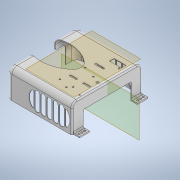
# Autodesk Inventor part: Enclosure
Saved by Autodesk Inventor 2020 (Build 240168000, 168)
## iProperties
Created: 2020-02-08
Part Number: Enclosure
Material: Generic
Document SubType Name: Modeling
Designer: pp445
Density: 1 g/cm^3
Appearance: Default
Author: pp445
Autodesk Inventor part; units mm, degrees
ref_plane "YZ Plane" through (0, 0, 0) normal (1, 0, 0) x (0, 1, 0)
ref_plane "XZ Plane" through (0, 0, 0) normal (0, 1, 0) x (-1, 0, 0)
ref_plane "XY Plane" through (0, 0, 0) normal (0, 0, 1) x (1, 0, 0)
sketch "Sketch1" plane through (0, 0, 0) normal (0, 1, 0) x (-1, 0, 0)
  line L0 (0, 0) -> (81, 0)
  line L1 (81, 0) -> (81, -120)
  line L2 (81, -120) -> (0, -120)
  line L3 (0, -120) -> (0, 0)
  line L4 (217, 28.5) -> (81, 28.5)
  line L5 (81, 28.5) -> (81, -146)
  line L6 (81, -146) -> (217, -146)
  line L7 (217, -146) -> (217, 28.5)
  line L8 (81, -60) -> (0, -60) construction
  point P0 (81, 0)
  point P1 (81, -120)
  dimension "d0" = 120
  dimension "d1" = 81
  dimension "d2" = 174.5
  dimension "d4" = 136
  dimension "d40" = 26
  constraints: 18 end point, 4 parallel, 2 horizontal, 2 perpendicular, 1 collinear, 1 midpoint, 1 point on line
  measures "d0" distance of L2.end L0.start
  measures "d1" distance of L0.start L0.end
  measures "d2" distance between parallel lines of L6 L4
  measures "d4" distance of L4.start L4.end
  measures "d40" distance between parallel lines of L2 L6
extrude "Extrusion1" add sketch "Sketch1" against normal blind 70
shell "Shell1" thickness 1.25 removed faces 3 at (-171.6667, -70, -39.1667) at (0, -23.3333, -40) at (-217, -23.3333, -87.8333)
sketch "Sketch3" plane through (0, -70, 0) normal (0, -1, 0) x (1, 0, 0)
  line L0 (-81, -146) -> (-81, -120) projected
  line L1 (0, -1.25) -> (0, 0) projected
  line L2 (0, 0) -> (-81, 0)
  line L3 (-81, -120) -> (0, -120) projected
  line L4 (0, -120) -> (-81, -120)
  line L5 (-81, -120) -> (-81, -146)
  line L6 (-81, -146) -> (0, -146)
  line L7 (0, -146) -> (0, -120)
  line L8 (-81, 0) -> (-81, 28.5) projected
  line L9 (-81, 0) -> (0, 0) projected
  line L10 (-217, 28.5) -> (-81, 28.5) projected
  line L11 (0, 0) -> (-81, 0)
  line L12 (-81, 0) -> (-81, 28.5)
  line L13 (-81, 28.5) -> (0, 28.5)
  line L14 (0, 28.5) -> (0, 0)
  constraints: 18 end point, 4 parallel, 3 horizontal, 2 perpendicular
extrude "Extrusion3" add sketch "Sketch3" against normal blind 3.175
sketch "Sketch5" plane through (0, -66.825, 0) normal (0, 1, 0) x (1, 0, 0)
  line L0 (0, 120) -> (0, 146) projected
  line L1 (0, 146) -> (-81, 146) projected
  line L2 (-81, 120) -> (-81, 146) projected
  line L3 (0, 120) -> (-81, 120) projected
  line L4 (-81, 0) -> (0, 0) projected
  line L5 (-81, -28.5) -> (-81, 0) projected
  line L6 (-81, -28.5) -> (0, -28.5) projected
  line L7 (0, -28.5) -> (0, 0) projected
  line L8 (0, 146) -> (0, 118.75) projected
  line L9 (-81, 120) -> (-81, 146) projected
  line L10 (0, 1.25) -> (0, -28.5) projected
  line L11 (0, -14.25) -> (-81, -14.25) construction
  line L12 (-81, -28.5) -> (-81, 0) projected
  circle A0 centre (-20.7, -14.25) radius 2.3813
  circle A1 centre (-46.1, -14.25) radius 2.3813
  circle A2 centre (-71.5, -14.25) radius 2.3813
  circle A3 centre (-20.7, 133.3) radius 2.3813
  circle A4 centre (-46.1, 133.3) radius 2.3813
  circle A5 centre (-71.5, 133.3) radius 2.3813
  line L13 (-81, 133.3) -> (0, 133.3) construction
  dimension "d18" = 20.7
  dimension "d19" = 25.4
  dimension "d20" = 25.4
  dimension "d21" = 4.7625
  dimension "d22" = 4.7625
  dimension "d23" = 4.7625
  dimension "d41" = 4.7625
  dimension "d42" = 4.7625
  dimension "d43" = 4.7625
  dimension "d44" = 20.7
  dimension "d45" = 25.4
  dimension "d46" = 25.4
  dimension "d47" = 13.3
  constraints: 9 point on line, 6 centre point, 4 end point, 1 midpoint, 1 perpendicular
  measures "d18" distance from line of L7 A0.centre
  measures "d19" distance of A0.centre A1.centre
  measures "d20" distance of A1.centre A2.centre
  measures "d21" diameter of A0
  measures "d22" diameter of A1
  measures "d23" diameter of A2
  measures "d41" diameter of A3
  measures "d42" diameter of A4
  measures "d43" diameter of A5
  measures "d44" distance from line of L8 A3.centre
  measures "d45" distance of A3.centre A4.centre
  measures "d46" distance of A4.centre A5.centre
  measures "d47" distance between parallel lines of L3 L13
extrude "Extrusion4" cut sketch "Sketch5" against normal up to surface (3.175 mm away) contours A3 | A4 | A5
ref_plane "Work Plane1" through (0, -1.25, -60) normal (0, 0, -1) x (-1, 0, 0)
mirror "Mirror1" about plane through (0, -1.25, -60) normal (0, 0, -1) of "Extrusion4"
mirror "Mirror2" about plane through (0, -1.25, -60) normal (0, 0, -1) of "Extrusion4"
sketch "Sketch9" plane through (0, 0, 0) normal (1, 0, 0) x (0, 0, -1)
  line L0 (1.25, -70) -> (1.25, -1.25) projected
  line L1 (1.25, -1.25) -> (118.75, -1.25) projected
  line L2 (118.75, -1.25) -> (118.75, -70) projected
  line L3 (146, -70) -> (118.75, -70) projected
  line L4 (146, -70) -> (146, -66.825) projected
  line L5 (120, -66.825) -> (146, -66.825) projected
  line L6 (120, 0) -> (120, -66.825) projected
  line L7 (0, 0) -> (120, 0) projected
  line L8 (0, 0) -> (0, -66.825) projected
  line L9 (-28.5, -66.825) -> (0, -66.825) projected
  line L10 (-28.5, -70) -> (-28.5, -66.825) projected
  line L11 (1.25, -70) -> (-28.5, -70) projected
extrude "Extrusion8" cut sketch "Sketch9" against normal blind 10
sketch "Sketch10" plane through (-10, 0, 0) normal (1, 0, 0) x (0, 0, -1)
  line L0 (1.25, -70) -> (-28.5, -70) projected
  line L1 (1.25, -1.25) -> (1.25, -70) projected
  line L2 (118.75, -1.25) -> (1.25, -1.25) projected
  line L3 (118.75, -70) -> (118.75, -1.25) projected
  line L4 (146, -70) -> (118.75, -70) projected
  line L5 (146, -66.825) -> (146, -70) projected
  line L6 (120, -66.825) -> (146, -66.825) projected
  line L7 (120, 0) -> (120, -66.825) projected
  line L8 (0, 0) -> (120, 0) projected
  line L9 (0, -66.825) -> (0, 0) projected
  line L10 (-28.5, -66.825) -> (0, -66.825) projected
  line L11 (-28.5, -70) -> (-28.5, -66.825) projected
  line L12 (1.25, -70) -> (-28.5, -70) projected
  line L13 (-28.5, -66.825) -> (-24.5, -66.825)
  line L14 (-24.5, -66.825) -> (-24.5, -70)
  line L15 (-24.5, -70) -> (-28.5, -70)
  line L16 (-28.5, -70) -> (-28.5, -66.825)
  dimension "d50" = 4
  constraints: 8 end point, 2 parallel, 1 horizontal, 1 perpendicular, 1 point on line
  measures "d50" distance between parallel lines of L11 L14
extrude "Extrusion9" cut sketch "Sketch10" against normal up to surface (71 mm away) contours L0 L11 L10 L14
pattern_linear "Rectangular Pattern2" count 2 spacing 7 along (0, 0, -1) count 2 spacing 7 along (0, 0, 1) of "Extrusion4"
mirror "Mirror3" about plane through (0, -1.25, -60) normal (0, 0, -1) of "Extrusion4", "Rectangular Pattern2"
sketch "Sketch11" plane through (-81, -70, 28.5) normal (0, 0, 1) x (1, 0, 0)
  line L0 (0, 70) -> (0, 0) projected
  line L1 (-136, 70) -> (0, 70) projected
  line L2 (0, 0) -> (-136, 0) projected
  line L3 (-1.25, 0) -> (-114, 0) projected
  line L4 (-3.175, 0) -> (-109.175, 0)
  line L5 (-109.175, 0) -> (-109.175, 58.175)
  line L6 (-109.175, 58.175) -> (-3.175, 58.175)
  line L7 (-3.175, 58.175) -> (-3.175, 0)
  line L8 (-95.5478, 52.5) -> (-95.5478, 7.5)
  circle A0 centre (-79.7364, 30) radius 27.5 construction
  arc A1 (-95.5478, 52.5) -> (-95.5478, 7.5) centre (-79.7364, 30) ccw
  line L9 (-56.175, 58.175) -> (-56.175, 0) construction
  line L10 (-16.8022, 52.5) -> (-16.8022, 7.5)
  circle A2 centre (-32.6136, 30) radius 27.5 construction
  arc A3 (-16.8022, 7.5) -> (-16.8022, 52.5) centre (-32.6136, 30) ccw
  line L11 (-79.7364, 30) -> (-32.6136, 30) construction
  line L12 (-93.0078, 54) -> (-80.3078, 54)
  line L13 (-80.3078, 54) -> (-80.3078, 6)
  line L14 (-80.3078, 6) -> (-93.0078, 6)
  line L15 (-93.0078, 6) -> (-93.0078, 54)
  line L16 (-93.0078, 30) -> (-80.3078, 30) construction
  line L17 (-77.7678, 54) -> (-65.0678, 54)
  line L18 (-65.0678, 54) -> (-65.0678, 6)
  line L19 (-65.0678, 6) -> (-77.7678, 6)
  line L20 (-77.7678, 6) -> (-77.7678, 54)
  line L21 (-62.5278, 54) -> (-49.8278, 54)
  line L22 (-49.8278, 54) -> (-49.8278, 6)
  line L23 (-49.8278, 6) -> (-62.5278, 6)
  line L24 (-62.5278, 6) -> (-62.5278, 54)
  line L25 (-47.2878, 54) -> (-34.5878, 54)
  line L26 (-34.5878, 54) -> (-34.5878, 6)
  line L27 (-34.5878, 6) -> (-47.2878, 6)
  line L28 (-47.2878, 6) -> (-47.2878, 54)
  line L29 (-32.0478, 54) -> (-19.3478, 54)
  line L30 (-19.3478, 54) -> (-19.3478, 6)
  line L31 (-19.3478, 6) -> (-32.0478, 6)
  line L32 (-32.0478, 6) -> (-32.0478, 54)
  line L33 (-136, 70) -> (-136, 0) projected
  point P0 (81, 70)
  point P1 (-65.0678, 30)
  point P2 (-77.7678, 30)
  point P3 (-49.8278, 30)
  point P4 (-62.5278, 30)
  point P5 (-34.5878, 30)
  point P6 (-47.2878, 30)
  point P7 (-19.3478, 30)
  point P8 (-32.0478, 30)
  dimension "d59" = 3.175
  dimension "d60" = 106
  dimension "d61" = 58.175
  dimension "d62" = 45
  dimension "d63" = 55
  dimension "d64" = 30
  dimension "d66" = 29.4386
  dimension "d70" = 48
  dimension "d71" = 2.54
  dimension "d72" = 12.7
  dimension "d83" = 15.24
  constraints: 58 end point, 8 point on circle, 4 centre point, 4 horizontal, 4 midpoint, 4 parallel, 4 symmetric about line, 3 perpendicular, 2 coincident, 1 collinear, 1 point on line, 1 vertical, 42 other
  measures "d59" distance between parallel lines of L0 L7
  measures "d60" distance of L5.end L6.end
  measures "d61" distance of L4.end L5.end
  measures "d62" distance of L8.start L8.end
  measures "d63" diameter of A0
  measures "d64" distance from line of L2 A0.centre
  measures "d66" distance from line of L5 A0.centre
  measures "d70" distance of L12.end L13.end
  measures "d71" distance between parallel lines of L8 L15
  measures "d72" distance between parallel lines of L15 L13
  measures "d83" distance of L12.start L17.start
extrude "Extrusion10" cut sketch "Sketch11" against normal up to surface (174.5 mm away) contours L8 A1 | A3 L10 | L12 L13 L14 L15 | L17 L18 L19 L20 | L21 L22 L23 L24 | L25 L26 L27 L28 | L29 L30 L31 L32
fillet "Fillet1" radius 2.54 8 edges at (-176.5478, -17.5, 27.875) (-176.5478, -62.5, 27.875) (-97.8022, -17.5, 27.875) (-97.8022, -62.5, 27.875) (-97.8022, -17.5, -145.375) (-97.8022, -62.5, -145.375) (-176.5478, -62.5, -145.375) (-176.5478, -17.5, -145.375)
fillet "Fillet2" radius 6.35 40 edges at (-174.0078, -64, 27.875) (-161.3078, -64, 27.875) (-161.3078, -16, 27.875) (-174.0078, -16, 27.875) (-158.7678, -64, 27.875) (-143.5278, -64, 27.875) (-128.2878, -64, 27.875) (-113.0478, -64, 27.875) (-100.3478, -64, 27.875) (-115.5878, -64, 27.875) (-130.8278, -64, 27.875) (-146.0678, -64, 27.875) (-158.7678, -16, 27.875) (-143.5278, -16, 27.875) (-128.2878, -16, 27.875) (-113.0478, -16, 27.875) (-100.3478, -16, 27.875) (-115.5878, -16, 27.875) (-130.8278, -16, 27.875) (-146.0678, -16, 27.875) (-174.0078, -16, -145.375) (-158.7678, -16, -145.375) (-143.5278, -16, -145.375) (-128.2878, -16, -145.375) (-113.0478, -16, -145.375) (-100.3478, -16, -145.375) (-115.5878, -16, -145.375) (-130.8278, -16, -145.375) (-146.0678, -16, -145.375) (-161.3078, -16, -145.375) (-100.3478, -64, -145.375) (-115.5878, -64, -145.375) (-130.8278, -64, -145.375) (-146.0678, -64, -145.375) (-161.3078, -64, -145.375) (-174.0078, -64, -145.375) (-158.7678, -64, -145.375) (-143.5278, -64, -145.375) (-128.2878, -64, -145.375) (-113.0478, -64, -145.375)
sketch "Sketch12" plane through (-10, 0, 0) normal (1, 0, 0) x (0, 0, -1)
  line L0 (-24.5, -66.825) -> (-24.5, -70) projected
  line L1 (1.25, -70) -> (-24.5, -70) projected
  line L2 (1.25, -1.25) -> (1.25, -70) projected
  line L3 (118.75, -1.25) -> (1.25, -1.25) projected
  line L4 (118.75, -70) -> (118.75, -1.25) projected
  line L5 (146, -70) -> (118.75, -70) projected
  line L6 (146, -66.825) -> (146, -70) projected
  line L7 (120, -66.825) -> (146, -66.825) projected
  line L8 (120, 0) -> (120, -66.825) projected
  line L9 (0, 0) -> (120, 0) projected
  line L10 (0, -66.825) -> (0, 0) projected
  line L11 (-24.5, -66.825) -> (0, -66.825) projected
  line L12 (0, -66.825) -> (0, 0) projected
  line L13 (1.25, -70) -> (0, -70)
  line L14 (0, -70) -> (0, 0)
  line L15 (0, 0) -> (1.25, 0)
  line L16 (1.25, 0) -> (1.25, -70)
  line L17 (118.75, -70) -> (144.75, -70) projected
  line L18 (120, 0) -> (120, -66.825) projected
  line L19 (118.75, -70) -> (120, -70)
  line L20 (120, -70) -> (120, 0)
  line L21 (120, 0) -> (118.75, 0)
  line L22 (118.75, 0) -> (118.75, -70)
  line L23 (118.75, 0) -> (1.25, 0)
  line L24 (1.25, 0) -> (1.25, -1.25)
  line L25 (1.25, -1.25) -> (118.75, -1.25)
  line L26 (118.75, -1.25) -> (118.75, 0)
  constraints: 24 end point, 6 parallel, 3 horizontal, 3 perpendicular
extrude "Extrusion11" cut sketch "Sketch12" against normal up to surface (72.25 mm away) contours L10 L9 L16 L2 L1 L14 | L9 L22 L3 L16 | L9 L8 L20 L5 L4 L22
sketch "Sketch13" plane through (-82.25, -1.25, -120) normal (1, 0, 0) x (0, 0, -1)
  line L0 (-120, 1.25) -> (0, 1.25) projected
  line L1 (-120, 0) -> (0, 0) projected
  line L2 (0, 1.25) -> (0, 0) projected
  line L3 (-120, 1.25) -> (0, 1.25) projected
  line L4 (-120, 0) -> (-120, 1.25) projected
  line L5 (0, 1.25) -> (-120, 1.25)
  line L6 (-120, 1.25) -> (-120, -26.75)
  line L7 (-120, -26.75) -> (0, -26.75)
  line L8 (0, -26.75) -> (0, 1.25)
  point P0 (-120, 1.25)
  point P1 (-120, 0)
  dimension "d90" = 28
  constraints: 8 end point, 2 parallel, 1 horizontal, 1 perpendicular
  measures "d90" distance between parallel lines of L0 L7
extrude "Extrusion12" add sketch "Sketch13" along normal up to surface (1.25 mm away)
fillet "Fillet6" radius 12.7 4 edges at (-149, 0, 28.5) (-149, 0, -146) (-149.625, -1.25, 27.25) (-149.625, -1.25, -144.75)
fillet "Fillet7" radius 3.175 10 edges at (-81, -3.7197, -142.2803) (-81, -39.7625, -146) (-81, -3.7197, 24.7803) (-81, -41.35, 28.5) (-81, 0, -58.75) (-82.25, -4.9697, -141.0303) (-82.25, -41.975, -144.75) (-82.25, -4.9697, 23.5303) (-82.25, -41.975, 27.25) (-82.25, -1.25, -58.75)
fillet "Fillet8" radius 3.175 3 edges at (-81, -66.825, 12.25) (-81.9299, -66.825, -145.0701) (-81, -66.825, -131.4125)
sketch "Sketch14" plane through (0, 0, 0) normal (0, 1, 0) x (1, 0, 0)
  line L0 (-125.838, 60) -> (-143.11, 60) construction
  line L1 (-152, 60) -> (-93.7, 60) construction
  line L2 (-143.3307, -3.1) -> (-126.0587, -3.1)
  line L3 (-126.0587, -3.1) -> (-126.0587, 9.6)
  line L4 (-126.0587, 9.6) -> (-143.3307, 9.6)
  line L5 (-143.3307, 9.6) -> (-143.3307, -3.1)
  circle A0 centre (-147.3307, 7.85) radius 1.75
  circle A1 centre (-122.0587, -1.35) radius 1.75
  line L6 (-110.337, -3.1) -> (-93.065, -3.1)
  line L7 (-93.065, -3.1) -> (-93.065, 9.6)
  line L8 (-93.065, 9.6) -> (-110.337, 9.6)
  line L9 (-110.337, 9.6) -> (-110.337, -3.1)
  circle A2 centre (-114.337, 7.85) radius 1.75
  circle A3 centre (-89.065, -1.35) radius 1.75
  line L10 (-136.9807, 53.65) -> (-115.2129, 53.65)
  line L11 (-115.2129, 53.65) -> (-115.2129, 66.35)
  line L12 (-115.2129, 66.35) -> (-136.9807, 66.35)
  line L13 (-136.9807, 66.35) -> (-136.9807, 53.65)
  circle A4 centre (-111.2129, 55.4) radius 1.75
  circle A5 centre (-140.9807, 64.6) radius 1.75
  line L14 (-146.5057, 60) -> (-84.175, 60) construction
  line L15 (-136.9807, 60) -> (-115.2129, 60) construction
  circle A6 centre (-93.065, 47.7) radius 3.25
  line L16 (-108.525, 102.85) -> (-100.375, 102.85)
  line L17 (-100.375, 102.85) -> (-100.375, 107.9)
  line L18 (-100.375, 107.9) -> (-108.525, 107.9)
  line L19 (-108.525, 107.9) -> (-108.525, 102.85)
  circle A7 centre (-96.875, 105.375) radius 2
  line L20 (-108.525, 105.375) -> (-100.375, 105.375) construction
  line L21 (-143.3307, 26.9) -> (-126.0587, 26.9)
  line L22 (-126.0587, 26.9) -> (-126.0587, 30.9)
  line L23 (-126.0587, 30.9) -> (-143.3307, 30.9)
  line L24 (-143.3307, 30.9) -> (-143.3307, 26.9)
  line L25 (-110.337, 26.9) -> (-93.065, 26.9)
  line L26 (-93.065, 26.9) -> (-93.065, 30.9)
  line L27 (-93.065, 30.9) -> (-110.337, 30.9)
  line L28 (-110.337, 30.9) -> (-110.337, 26.9)
  line L29 (-136.9807, 83.65) -> (-115.2129, 83.65)
  line L30 (-115.2129, 83.65) -> (-115.2129, 87.65)
  line L31 (-115.2129, 87.65) -> (-136.9807, 87.65)
  line L32 (-136.9807, 87.65) -> (-136.9807, 83.65)
  line L33 (-124.985, 109.185) -> (-94.985, 109.185)
  line L34 (-94.985, 109.185) -> (-94.985, 120.685)
  line L35 (-94.985, 120.685) -> (-124.985, 120.685)
  line L36 (-124.985, 120.685) -> (-124.985, 109.185)
  line L37 (-92.875, 99.946) -> (-92.875, 129.6859) construction
  line L38 (-217, 133.3) -> (-84.175, 133.3) projected
  line L39 (-84.175, -15.8) -> (-217, -15.8) projected
  line L40 (-84.175, 133.3) -> (-84.175, -15.8) projected
  line L41 (-217, 133.3) -> (-217, -15.8) projected
  point P0 (0, 0)
  dimension "d107" = 17.272
  dimension "d108" = 12.7
  dimension "d109" = 3.5
  dimension "d110" = 3.5
  dimension "d111" = 4
  dimension "d112" = 4
  dimension "d114" = 17.272
  dimension "d115" = 12.7
  dimension "d120" = 3.5
  dimension "d121" = 3.5
  dimension "d122" = 4
  dimension "d123" = 4
  dimension "d128" = 21.7678
  dimension "d129" = 12.7
  dimension "d130" = 3.5
  dimension "d131" = 3.5
  dimension "d132" = 4
  dimension "d133" = 4
  dimension "d135" = 6.5
  dimension "d137" = 38.1
  dimension "d146" = 5.05
  dimension "d147" = 8.15
  dimension "d148" = 4
  dimension "d149" = 3.5
  dimension "d152" = 17.272
  dimension "d153" = 4
  dimension "d154" = 30
  dimension "d155" = 17.272
  dimension "d156" = 4
  dimension "d157" = 30
  dimension "d158" = 21.7678
  dimension "d159" = 4
  dimension "d160" = 30
  dimension "d164" = 11.5
  dimension "d165" = 30
  dimension "d166" = 3.81
  dimension "d167" = 4
  dimension "d168" = 2.11
  constraints: 76 end point, 17 parallel, 9 horizontal, 8 centre point, 8 perpendicular, 6 tangent, 4 midpoint, 4 point on line, 3 collinear
  measures "d107" distance of L2.start L2.end
  measures "d108" distance of L2.end L3.end
  measures "d109" diameter of A1
  measures "d110" diameter of A0
  measures "d111" distance from line of L3 A1.centre
  measures "d112" distance from line of L5 A0.centre
  measures "d114" distance of L6.start L6.end
  measures "d115" distance of L6.end L7.end
  measures "d120" diameter of A3
  measures "d121" diameter of A2
  measures "d122" distance from line of L7 A3.centre
  measures "d123" distance from line of L9 A2.centre
  measures "d128" distance of L10.start L10.end
  measures "d129" distance of L10.end L11.end
  measures "d130" diameter of A4
  measures "d131" diameter of A5
  measures "d132" distance from line of L11 A4.centre
  measures "d133" distance from line of L13 A5.centre
  measures "d135" diameter of A6
  measures "d137" distance from line of L8 A6.centre
  measures "d146" distance of L16.end L17.end
  measures "d147" distance of L17.end L18.end
  measures "d148" diameter of A7
  measures "d149" distance from line of L17 A7.centre
  measures "d152" distance of L21.start L21.end
  measures "d153" distance of L23.end L21.start
  measures "d154" distance between parallel lines of L2 L21
  measures "d155" distance of L25.start L25.end
  measures "d156" distance of L27.end L25.start
  measures "d157" distance between parallel lines of L6 L25
  measures "d158" distance of L29.start L29.end
  measures "d159" distance of L31.end L29.start
  measures "d160" distance between parallel lines of L10 L29
  measures "d164" distance of L33.end L34.end
  measures "d165" distance of L34.end L35.end
  measures "d166" distance from line of A7.centre L33
  measures "d167" distance from line of A7.centre L37
  measures "d168" distance between parallel lines of L37 L34
extrude "Extrusion13" cut sketch "Sketch14" against normal up to surface (1.25 mm away) contours A0 | A1 | A2 | A3 | A4 | A5 | A6 | A7 | L24 L23 L22 L21 | L28 L27 L26 L25 | L32 L31 L30 L29 | L36 L35 L34 L33
ref_plane "Work Plane2" through (0, 12, 0) normal (0, 1, 0) x (1, 0, 0)
sketch "Sketch16" plane through (-10, 0, 0) normal (1, 0, 0) x (0, 0, -1)
  line L0 (0, -70) -> (0, -66.825) projected
  line L1 (-24.5, -66.825) -> (0, -66.825) projected
  line L2 (-24.5, -66.825) -> (-24.5, -70) projected
  line L3 (0, -70) -> (-24.5, -70) projected
  line L4 (120, -66.825) -> (120, -70) projected
  line L5 (146, -70) -> (120, -70) projected
  line L6 (146, -66.825) -> (146, -70) projected
  line L7 (120, -66.825) -> (146, -66.825) projected
  point P0 (0, 0)
extrude "Extrusion14" cut sketch "Sketch16" against normal blind 55.88
sketch "Sketch17" plane through (-217, 0, -133.3) normal (-1, 0, 0) x (0, 0, 1)
  arc A0 (0, 0) -> (-12.7, -12.7) centre (0, -12.7) ccw projected
  line L0 (-12.7, -12.7) -> (-12.7, -70) projected
  line L1 (-11.45, -70) -> (-12.7, -70) projected
  line L2 (-11.45, -70) -> (-11.45, -13.95) projected
  arc A1 (1.25, -1.25) -> (-11.45, -13.95) centre (1.25, -13.95) ccw projected
  line L3 (1.25, -1.25) -> (147.85, -1.25) projected
  arc A2 (160.55, -13.95) -> (147.85, -1.25) centre (147.85, -13.95) ccw projected
  line L4 (160.55, -13.95) -> (160.55, -70) projected
  line L5 (161.8, -70) -> (160.55, -70) projected
  line L6 (161.8, -12.7) -> (161.8, -70) projected
  arc A3 (161.8, -12.7) -> (149.1, 0) centre (149.1, -12.7) ccw projected
  line L7 (0, 0) -> (149.1, 0) projected
  point P0 (133.3, 0)
extrude "Extrusion15" add sketch "Sketch17" along normal blind 25
sketch "Sketch18" plane through (-242, 0, -133.3) normal (-1, 0, 0) x (0, 0, 1)
  line L0 (1.25, -1.25) -> (147.85, -1.25) projected
  arc A0 (160.55, -13.95) -> (147.85, -1.25) centre (147.85, -13.95) ccw projected
  line L1 (160.55, -13.95) -> (160.55, -70) projected
  line L2 (160.55, -70) -> (161.8, -70) projected
  line L3 (161.8, -70) -> (161.8, -12.7) projected
  arc A1 (161.8, -12.7) -> (149.1, 0) centre (149.1, -12.7) ccw projected
  line L4 (149.1, 0) -> (0, 0) projected
  arc A2 (0, 0) -> (-12.7, -12.7) centre (0, -12.7) ccw projected
  line L5 (-12.7, -12.7) -> (-12.7, -70) projected
  line L6 (-12.7, -70) -> (-11.45, -70) projected
  line L7 (-11.45, -70) -> (-11.45, -13.95) projected
  arc A3 (1.25, -1.25) -> (-11.45, -13.95) centre (1.25, -13.95) ccw projected
  line L8 (1.25, -1.25) -> (147.85, -1.25) projected
  line L9 (-11.45, -70) -> (-11.45, -13.95) projected
  line L10 (-11.45, -26.25) -> (160.55, -26.25)
  line L11 (160.55, -13.95) -> (160.55, -70) projected
  line L12 (-11.45, -26.25) -> (16.55, -26.25)
  line L13 (16.55, -26.25) -> (16.55, -70)
  line L14 (16.55, -70) -> (-11.45, -70)
  line L15 (-11.45, -70) -> (-11.45, -26.25)
  line L16 (160.55, -70) -> (132.55, -70)
  line L17 (132.55, -70) -> (132.55, -26.25)
  line L18 (132.55, -26.25) -> (160.55, -26.25)
  line L19 (160.55, -26.25) -> (160.55, -70)
  line L20 (-12.7, -70) -> (-11.45, -70) projected
  point P0 (133.3, 0)
  point P1 (16.55, -26.25)
  dimension "d176" = 25
  dimension "d177" = 28
  dimension "d178" = 28
  constraints: 18 end point, 4 parallel, 3 perpendicular, 3 point on line, 2 horizontal, 1 collinear
  measures "d176" distance between parallel lines of L0 L10
  measures "d177" distance between parallel lines of L7 L13
  measures "d178" distance between parallel lines of L1 L17
extrude "Extrusion16" add sketch "Sketch18" along normal blind 1.5
sketch "Sketch19" plane through (-84.175, -63.65, -146) normal (0, 0, -1) x (-1, 0, 0)
  line L0 (-18.295, -3.175) -> (-18.295, -6.35) projected
  line L1 (-18.295, -6.35) -> (159.325, -6.35) projected
  line L2 (159.325, 50.95) -> (159.325, -6.35) projected
  line L3 (0, 50.95) -> (159.325, 50.95) projected
  line L4 (0, 0) -> (0, 50.95) projected
  line L5 (-18.295, -3.175) -> (-5.4993, -3.175) projected
  line L6 (31.4128, 6) -> (31.4128, 41.3) projected
  arc A0 (44.1128, 41.3) -> (31.4128, 41.3) centre (37.7628, 41.3) ccw projected
  line L7 (44.1128, 41.3) -> (44.1128, 6) projected
  arc A1 (31.4128, 6) -> (44.1128, 6) centre (37.7628, 6) ccw projected
  arc A2 (61.8928, 6) -> (74.5928, 6) centre (68.2428, 6) ccw projected
  line L8 (61.8928, 6) -> (61.8928, 41.3) projected
  arc A3 (74.5928, 41.3) -> (61.8928, 41.3) centre (68.2428, 41.3) ccw projected
  line L9 (74.5928, 41.3) -> (74.5928, 6) projected
  line L10 (77.1328, 6) -> (77.1328, 41.3) projected
  arc A4 (89.8328, 41.3) -> (77.1328, 41.3) centre (83.4828, 41.3) ccw projected
  line L11 (89.8328, 41.3) -> (89.8328, 6) projected
  arc A5 (77.1328, 6) -> (89.8328, 6) centre (83.4828, 6) ccw projected
  line L12 (13.6272, 40.5683) -> (13.6272, 6.7317) projected
  arc A6 (9.2197, 5.0101) -> (13.6272, 6.7317) centre (11.0872, 6.7317) ccw projected
  arc A7 (9.2197, 42.2899) -> (9.2197, 5.0101) centre (29.4386, 23.65) ccw projected
  arc A8 (13.6272, 40.5683) -> (9.2197, 42.2899) centre (11.0872, 40.5683) ccw projected
  arc A9 (59.3528, 41.3) -> (46.6528, 41.3) centre (53.0028, 41.3) ccw projected
  line L13 (59.3528, 41.3) -> (59.3528, 6) projected
  arc A10 (46.6528, 6) -> (59.3528, 6) centre (53.0028, 6) ccw projected
  line L14 (46.6528, 6) -> (46.6528, 41.3) projected
  line L15 (28.8728, 41.3) -> (28.8728, 6) projected
  arc A11 (16.1728, 6) -> (28.8728, 6) centre (22.5228, 6) ccw projected
  line L16 (16.1728, 6) -> (16.1728, 41.3) projected
  arc A12 (28.8728, 41.3) -> (16.1728, 41.3) centre (22.5228, 41.3) ccw projected
  line L17 (92.3728, 6.7317) -> (92.3728, 40.5683) projected
  arc A13 (96.7803, 42.2899) -> (92.3728, 40.5683) centre (94.9128, 40.5683) ccw projected
  arc A14 (96.7803, 5.0101) -> (96.7803, 42.2899) centre (76.5614, 23.65) ccw projected
  arc A15 (92.3728, 6.7317) -> (96.7803, 5.0101) centre (94.9128, 6.7317) ccw projected
  line L18 (-18.295, -6.35) -> (159.325, -6.35) projected
  line L19 (106.325, -6.35) -> (141.325, -6.35)
  line L20 (141.325, -6.35) -> (141.325, 8.65)
  line L21 (141.325, 8.65) -> (106.325, 8.65)
  line L22 (106.325, 8.65) -> (106.325, -6.35)
  point P0 (-84.175, 63.65)
  dimension "d181" = 18
  dimension "d182" = 35
  dimension "d183" = 15
  constraints: 8 end point, 2 parallel, 1 horizontal, 1 perpendicular, 1 point on line, 1 other
  measures "d181" distance between parallel lines of L2 L20
  measures "d182" distance between parallel lines of L20 L22
  measures "d183" distance between parallel lines of L1 L21
extrude "Extrusion17" cut sketch "Sketch19" against normal up to surface (1.25 mm away) contours L22 L21 L20 L1
fillet "Fillet9" radius 3.175 2 edges at (-190.5, -55, -145.375) (-225.5, -55, -145.375)
sketch "Sketch20" plane through (0, 0, 0) normal (0, 1, 0) x (1, 0, 0)
  line L0 (-84.175, 133.3) -> (-243.5, 133.3) projected
  line L1 (-243.5, -15.8) -> (-243.5, 133.3) projected
  line L2 (-84.175, -15.8) -> (-243.5, -15.8) projected
  line L3 (-84.175, 133.3) -> (-84.175, -15.8) projected
  line L4 (-77.825, 0) -> (-65.88, 0) projected
  line L5 (-65.88, 120) -> (-77.825, 120) projected
  line L6 (-65.88, 120) -> (-82.25, 120) projected
  line L7 (-65.88, 0) -> (-65.88, 120)
  line L8 (-65.88, 60) -> (-243.5, 60) construction
  circle A0 centre (-209.5, 60) radius 37
  circle A1 centre (-166.5, 60) radius 20
  line L9 (-153.5831, 44.7306) -> (-189.8532, 14.0486) construction
  line L10 (-153.5831, 44.7306) -> (-176.2501, 25.5558) construction
  line L11 (-176.2501, 25.5558) -> (-206.5324, 23.1192) construction
  spline S0 degree 2 poles (-153.5831, 44.7306) (-176.2501, 25.5558) (-206.5324, 23.1192) knots 1 1 1 2 2 2
  line L12 (-153.5831, 75.2694) -> (-176.2501, 94.4442) construction
  line L13 (-176.2501, 94.4442) -> (-206.5324, 96.8808) construction
  spline S1 degree 2 poles (-153.5831, 75.2694) (-176.2501, 94.4442) (-206.5324, 96.8808) knots 1 1 1 2 2 2
  line L14 (-212.4667, 23.1191) -> (-235.091, 24.8868) construction
  line L15 (-235.091, 24.8868) -> (-243.5, 29.3896) construction
  spline S2 degree 2 poles (-212.4667, 23.1191) (-235.091, 24.8868) (-243.5, 29.3896) knots 1 1 1 2 2 2
  line L16 (-212.4667, 96.8809) -> (-235.091, 95.1132) construction
  line L17 (-235.091, 95.1132) -> (-243.5, 90.6104) construction
  spline S3 degree 2 poles (-212.4667, 96.8809) (-235.091, 95.1132) (-243.5, 90.6104) knots 1 1 1 2 2 2
  point P0 (0, 0)
  point P1 (-206.5324, 96.8808)
  point P2 (-212.4667, 96.8809)
  dimension "d191" = 40
  dimension "d188" = 74
  dimension "d189" = 34
  dimension "d190" = 43
  dimension "d192" = 34.4442
  dimension "d193" = 9.7501
  dimension "d194" = 35.1132
  dimension "d195" = 25.591
  dimension "d196" = 30.6104
  dimension "d205" = 2.9667
  constraints: 6 end point, 6 symmetric about line, 5 point on line, 2 point on circle, 1 centre point, 1 midpoint, 1 perpendicular, 1 tangent, 1 vertical, 17 other
  measures "d188" diameter of A0
  measures "d189" distance from line of L1 A0.centre
  measures "d190" distance of A0.centre point (-166.5, 60)
  measures "d192" vertical distance of point (-166.5, 60) L10.end
  measures "d193" horizontal distance of point (-166.5, 60) L10.end
  measures "d194" vertical distance of A0.centre L14.end
  measures "d195" horizontal distance of A0.centre L14.end
  measures "d196" vertical distance of A0.centre L15.end
  measures "d205" horizontal distance of A0.centre L14.start
extrude "Extrusion18" cut sketch "Sketch20" against normal up to surface (1.25 mm away) contours S3 A0 L1 | A0 A1 L1 | L1 A0 S2 | S1 A1 A0 | A1 A0 | A0 A1 | A0 A1 S0
sketch "Sketch21" plane through (-243.5, 0, -133.3) normal (-1, 0, 0) x (0, 0, 1)
  line L0 (42.6896, -1.25) -> (42.6896, 0) projected
  line L1 (103.9104, -1.25) -> (42.6896, -1.25) projected
  line L2 (16.55, -26.25) -> (132.55, -26.25) projected
  line L3 (103.9104, 0) -> (103.9104, -1.25) projected
  line L4 (42.6896, -1.25) -> (42.6896, -26.25)
  line L5 (16.55, -26.25) -> (132.55, -26.25) projected
  line L6 (103.9104, -1.25) -> (103.9104, -26.25)
  point P0 (133.3, 0)
  constraints: 4 end point, 2 perpendicular, 2 point on line
extrude "Extrusion19" cut sketch "Sketch21" against normal up to surface (1.5 mm away)
fillet "Fillet10" radius 6.35 2 edges at (-242.75, -26.25, -116.75) (-242.75, -26.25, -0.75)
sketch "Sketch22" plane through (-243.5, -1.25, -90.6104) normal (0, 1, 0) x (1, 0, 0)
  line L0 (0, 0) -> (1.5, 0) projected
  line L1 (1.5, 0.7314) -> (1.5, 0) projected
  spline S0 degree 2 poles (0, 0) (0.7007, 0.3752) (1.5, 0.7314) knots 0 0 0 1 1 1 projected
  line L2 (1.5, -61.2208) -> (0, -61.2208) projected
  spline S1 degree 2 poles (1.5, -61.9522) (0.7007, -61.596) (0, -61.2208) knots 0 0 0 1 1 1 projected
  line L3 (1.5, -61.2208) -> (1.5, -61.9522) projected
  point P0 (243.5, -90.6104)
  constraints: 2 other
extrude "Extrusion20" cut sketch "Sketch22" against normal up to surface (25 mm away)
fillet "Fillet11" radius 12.7 12 edges at (-242, -4.9697, 23.5303) (-242, -1.25, -7.0541) (-242, -41.975, 27.25) (-243.5, 0, -6.7948) (-243.5, -41.35, 28.5) (-243.5, -3.7197, 24.7803) (-242, -1.25, -111.6959) (-242, -41.975, -144.75) (-242, -4.9697, -141.0303) (-243.5, -3.7197, -142.2803) (-243.5, -41.35, -146) (-243.5, 0, -111.9552)
fillet "Fillet12" radius 3.175 2 edges at (-242.7747, -26.25, -90.9808) (-242.7747, -26.25, -29.0192)
fillet "Fillet13" radius 3.175 2 edges at (-81.625, -28, 0) (-81.625, -28, -120)
equation "\"d20\" = d19"
equation "\"d22\" = d21"
equation "\"d23\" = d21"
equation "\"d41\" = d21"
equation "\"d42\" = d41"
equation "\"d43\" = d41"
equation "\"d44\" = d18"
equation "\"d45\" = d19"
equation "\"d46\" = d45"
body "Solid1"
